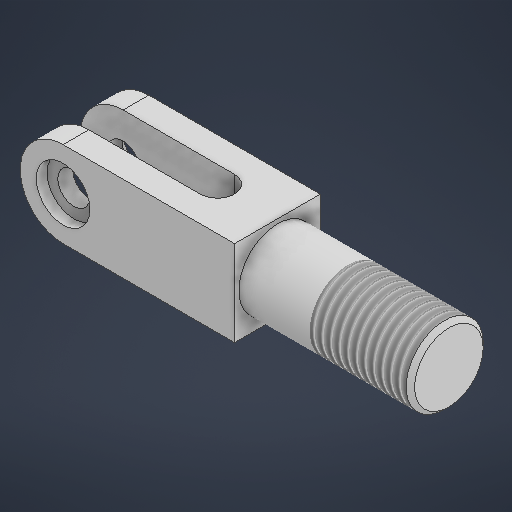
# Autodesk Inventor part: Partultimaparte
Saved by Autodesk Inventor 2026 (Build 300175050, 175E)
## iProperties
Created: 2026-04-09
Part Number: Partultimaparte
Material: Generic
Document SubType Name: Modeling
Designer: Administrator
Density: 1 g/cm^3
Appearance: Default
Author: Administrator
Autodesk Inventor part; units mm, degrees
ref_plane "YZ Plane" through (0, 0, 0) normal (1, 0, 0) x (0, 1, 0)
ref_plane "XZ Plane" through (0, 0, 0) normal (0, 1, 0) x (-1, 0, 0)
ref_plane "XY Plane" through (0, 0, 0) normal (0, 0, 1) x (1, 0, 0)
sketch "Sketch1" plane through (0, 0, 0) normal (0, 0, 1) x (1, 0, 0)
  line L0 (0, 0) -> (100, 0)
  line L1 (100, 0) -> (100, 40)
  line L2 (100, 40) -> (0, 40)
  line L3 (0, 40) -> (0, 0)
  dimension "d0" = 100
  dimension "d1" = 40
  constraints: 8 end point, 3 perpendicular, 1 horizontal
  measures "d0" distance between parallel lines of L1 L3
  measures "d1" distance between parallel lines of L0 L2
extrude "Extrusion1" add sketch "Sketch1" along normal mid plane 40
sketch "Sketch2" plane through (100, 0, 20) normal (1, 0, 0) x (0, 0, -1)
  line L0 (40, 40) -> (0, 40) projected
  circle A0 centre (20, 20) radius 18
  point P0 (20, 0)
  dimension "d5" = 36
  constraints: 1 centre point
  measures "d5" diameter of A0
extrude "Extrusion2" add sketch "Sketch2" along normal blind 80
thread "Thread1" size "M36x4" class "6g" standard "ANSI Metric M Profile" length 80 offset 33
chamfer "Chamfer1" distance 2 angle 45 1 edges at (180, 20, 18)
sketch "Sketch3" plane through (0, 0, 20) normal (0, 0, 1) x (1, 0, 0)
  line L0 (0, 0) -> (100, 0) projected
  line L1 (100, 40) -> (0, 40) projected
  circle A0 centre (20, 20) radius 7.5
  circle A1 centre (20, 20) radius 12.5
  line L2 (100, 0) -> (100, 40) projected
  dimension "d13" = 80
  dimension "d14" = 15
  dimension "d15" = 25
  constraints: 2 centre point, 1 coincident
  measures "d13" distance from line of L2 A0.centre
  measures "d14" diameter of A0
  measures "d15" diameter of A1
hole "Hole1" at (20, 20, 20) direction (0, 0, -1) diameter 15 end through all counterbore diameter 25 counterbore depth 5
fillet "Fillet1" radius 20 1 edges at (0, 40, 0)
fillet "Fillet2" radius 20 1 edges at (0, 0, 0)
sketch "Sketch9" plane through (100, 40, 20) normal (0, 1, 0) x (1, 0, 0)
  line L0 (0, 0) -> (-80, 0) projected
  line L1 (-28, 0) -> (-28, 39.5262)
  line L2 (0, 40) -> (0, 0) projected
  line L3 (-108, 28) -> (-28, 28)
  line L4 (-28, 28) -> (-28, 12)
  line L5 (-28, 12) -> (-108, 12)
  line L6 (-108, 12) -> (-108, 28)
  line L7 (-80, 40) -> (0, 40) projected
  circle A0 centre (-28, 20) radius 8
  point P0 (-100, 20)
  point P1 (-68, 12)
  point P2 (-28, 12)
  point P3 (-28, 28)
  dimension "d37" = 28
  dimension "d38" = 0
  dimension "d39" = 12
  dimension "d40" = 16
  dimension "d41" = 16
  dimension "d42" = 80
  dimension "d43" = 16
  constraints: 10 end point, 2 midpoint, 2 parallel, 1 centre point, 1 horizontal, 1 perpendicular, 1 point on line, 1 vertical
  measures "d37" distance between parallel lines of L1 L2
  measures "d38" distance between parallel lines of L4 L1
  measures "d39" distance between parallel lines of L7 L3
  measures "d40" distance from line of L3 point (-68, 12)
  measures "d41" distance of L5.end L3.start
  measures "d42" distance between parallel lines of L6 L1
  measures "d43" diameter of A0
extrude "Extrusion5" cut sketch "Sketch9" against normal blind 40
sketch "Sketch12" plane through (0, 0, -20) normal (0, 0, -1) x (-1, 0, 0)
  line L0 (-20, 0) -> (-100, 0) projected
  circle A0 centre (-20, 20) radius 12.5 projected
  circle A1 centre (-20, 20) radius 12.5
  point P0 (0, 0)
  constraints: 1 centre point, 1 coincident
extrude "Extrusion6" cut sketch "Sketch12" against normal blind 5
body "Solid1"
